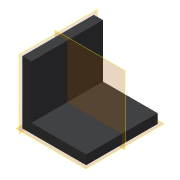
# Autodesk Inventor part: solid_base_feature
Saved by Autodesk Inventor 2022 Beta2 (Build 260130000, 130) ContinuousBuild 0
## iProperties
Shininess: 64.0
Length Units: 11272
Angle Units: 11279
Time Units: 11290
Mass Units: 11286
Length Display Precision: 3
Angle Display Precision: 2
Compacted: True
Part Number: solid_base_feature
Document SubType Name: Modeling
Created: 2004-02-27
Designer: mpaknia
Manufacturer: Standard
Standards Organization: Custom
Density: 11.37 g/cm^3
Material: Generic
Appearance: Generic
Density: 0.0
Volumn: 0.0
Area: 0.0
PropertySet Name: Model Information
Control State: 0
Master: False
Checked Out: False
Author: mpaknia
Autodesk Inventor part; units mm, degrees
sketch "Sketch1" plane through (0, 0, 0) normal (0, 0, 1) x (1, 0, 0)
  line L0 (0, 22.215) -> (0, 0)
  line L1 (0, 0) -> (22.6684, 0)
  line L2 (22.6684, 0) -> (22.6684, 3.3031)
  line L3 (22.6684, 3.3031) -> (3.2383, 3.3031)
  line L4 (3.2383, 3.3031) -> (3.2383, 22.215)
  line L5 (3.2383, 22.215) -> (0, 22.215)
  line L6 (0, 28.8795) -> (0, -2.2215) projected
  line L7 (-2.2668, 0) -> (29.4689, 0) projected
  constraints: 12 end point, 4 parallel, 2 collinear, 1 perpendicular, 1 vertical
extrude "Extrusion1" add sketch "Sketch1" along normal mid plane 25.4
body "Solid1"
